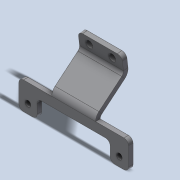
# Autodesk Inventor part: MuzzleHeadConnector2
Saved by Autodesk Inventor 2020 (Build 240168000, 168)
## iProperties
Created: 2021-07-22
Part Number: MuzzleHeadConnector2
Material: Generic
Document SubType Name: Sheet Metal
Designer: Val
Density: 1 g/cm^3
Sheet Metal Rule: Default
Appearance: Default
Flat Pattern Width: 5.75592 cm
Flat Pattern Length: 7.62 cm
Flat Pattern Area: 43.8601 cm^2
Sheet Metal Width: 2.266 in
Sheet Metal Length: 3.000 in
Sheet Metal Area: 6.798 in^2
Author: Val
Autodesk Inventor part; units mm, degrees
ref_plane "YZ Plane" through (0, 0, 0) normal (1, 0, 0) x (0, 1, 0)
ref_plane "XZ Plane" through (0, 0, 0) normal (0, 1, 0) x (-1, 0, 0)
ref_plane "XY Plane" through (0, 0, 0) normal (0, 0, 1) x (1, 0, 0)
sketch "Base" plane through (0, 0, 0) normal (0, 0, 1) x (1, 0, 0)
  line L0 (-38.1, 19.05) -> (38.1, 19.05)
  line L1 (38.1, 19.05) -> (38.1, 0)
  line L2 (38.1, 0) -> (-38.1, 0)
  line L3 (-38.1, 0) -> (-38.1, 19.05)
  line L4 (0, -3.81) -> (0, 22.86) construction
  line L5 (-25.4, 0) -> (-25.4, 12.7)
  line L6 (-25.4, 12.7) -> (25.4, 12.7)
  line L7 (25.4, 12.7) -> (25.4, 0)
  line L8 (-25.4, 12.7) -> (-38.1, 0) construction
  circle A0 centre (-31.75, 6.35) radius 2
  circle A1 centre (31.75, 6.35) radius 2
  point P0 (0, 0)
  point P1 (0, 19.05)
  dimension "d1" = 76.2
  dimension "d3" = 19.05
  dimension "d5" = 12.7
  dimension "d6" = 12.7
  dimension "d8" = 6.35
  dimension "d9" = 4
  measures "d1" distance of L0.start L0.end
  measures "d3" distance of L0.end L1.end
  measures "d5" distance between parallel lines of L3 L5
  measures "d6" distance between parallel lines of L1 L7
  measures "d8" distance between parallel lines of L0 L6
  measures "d9" diameter of A0
extrude "Plate1" add sketch "Base" along normal blind 3.175 contours L0 L1 L2 L7 L6 L5 L3
sketch "Sketch2" plane through (38.1, 21.4928, -1.1469) normal (0, 0.7693996, 0.6387678) x (-1, 0, 0)
  line L0 (76.2, 0) -> (0, 0)
  line L1 (0, 0) -> (0, -22.4187)
  line L2 (0, -22.4187) -> (76.2, -22.4187)
  line L3 (76.2, -22.4187) -> (76.2, 0)
  constraints: 6 end point, 1 horizontal, 1 perpendicular, 1 vertical
edge flange "MiddleFlangeFeature" height 25.4 angle 50.3 thickness 3.175 bend radius 3.175 thickness toward (0, 0.7693996, 0.6387678) relief straight relief width 3.175 relief depth 1.5875 edges at (0, 19.05, 0) wall of the first edge with corners at (-38.1, 21.4928, -1.1469) (38.1, 21.4928, -1.1469) (38.1, 35.8132, -18.3958) (-38.1, 35.8132, -18.3958)
bend "Bend1"
corner "Corner1"
sketch "Sketch3" plane through (38.1, 38.256, -16.3677) normal (0, 0.1166707, -0.9931706) x (-1, 0, 0)
  line L0 (76.2, 0) -> (0, 0)
  line L1 (0, 0) -> (0, -10.9761)
  line L2 (0, -10.9761) -> (76.2, -10.9761)
  line L3 (76.2, -10.9761) -> (76.2, 0)
  constraints: 6 end point, 1 horizontal, 1 perpendicular, 1 vertical
edge flange "MountFlangeFeature" height 12.7 angle -57 thickness 3.175 bend radius 3.175 thickness toward (0, 0.1166707, -0.9931706) relief straight relief width 3.175 relief depth 1.5875 edges at (0, 35.8132, -18.3958) wall of the first edge with corners at (-38.1, 38.256, -16.3677) (38.1, 38.256, -16.3677) (38.1, 49.1572, -15.0872) (-38.1, 49.1572, -15.0872)
bend "Bend2"
corner "Corner2"
sketch "TaperCut" plane through (0, 0, 3.175) normal (0, 0, 1) x (1, 0, 0)
  line L0 (-38.1, 19.05) -> (-38.1, 0) projected
  line L1 (-38.1, 19.05) -> (-15.24, 19.05)
  line L2 (-38.1, 19.05) -> (38.1, 19.05) projected
  line L3 (-15.24, 19.05) -> (-15.24, 49.1572)
  line L4 (-38.1, 39.9681) -> (-38.1, 49.1572) construction
  line L5 (-38.1, 49.1572) -> (38.1, 49.1572) projected
  line L6 (-38.1, 0) -> (-38.1, 19.05) projected
  line L7 (-38.1, 49.1572) -> (-38.1, 19.05)
  point P0 (0, 0)
  dimension "d35" = 22.86
  constraints: 6 end point, 2 point on line, 1 vertical
  measures "d35" distance between parallel lines of L4 L3
cut across bends "TaperCutFeature" sketch "TaperCut" k factor 0.44
mirror "TaperCutMirrorFeature" about plane through (0, 0, 0) normal (1, 0, 0) of "TaperCutFeature"
sketch "MountCut" plane through (-38.1, 49.1572, -15.0872) normal (0, -0.1166707, 0.9931706) x (1, 0, 0)
  line L0 (0, -8.402) -> (22.86, -8.402) projected
  line L1 (0, -8.402) -> (0, 0) projected
  line L2 (22.86, -8.402) -> (0, -8.402)
  line L3 (0, -8.402) -> (0, 0)
  line L4 (0, 0) -> (22.86, 0)
  line L5 (22.86, 0) -> (22.86, -8.402)
  line L6 (53.34, -8.402) -> (53.34, -9.2522) projected
  line L7 (53.34, -8.402) -> (76.2, -8.402)
  line L8 (76.2, -8.402) -> (76.2, 0)
  line L9 (76.2, 0) -> (53.34, 0)
  line L10 (53.34, 0) -> (53.34, -8.402)
  point P0 (38.1, -47.0612)
  constraints: 16 end point, 4 parallel, 2 horizontal, 2 perpendicular
extrude "MountCutFeature" cut sketch "MountCut" against normal blind 3.175
fillet "FilletsFeature" radius 3.175 10 edges at (-15.24, 49.3424, -16.6638) (15.24, 49.3424, -16.6638) (-38.1, 19.05, 1.5875) (-38.1, 0, 1.5875) (38.1, 19.05, 1.5875) (38.1, 0, 1.5875) (25.4, 0, 1.5875) (25.4, 12.7, 1.5875) (-25.4, 0, 1.5875) (-25.4, 12.7, 1.5875)
sketch "MountHoles" plane through (-38.1, 49.1572, -15.0872) normal (0, -0.1166707, 0.9931706) x (1, 0, 0)
  line L0 (0, 0) -> (76.2, 0) projected
  line L1 (38.1, 0) -> (38.1, -9.2522) construction
  line L2 (0, -9.2522) -> (76.2, -9.2522) projected
  circle A0 centre (30.1, -4.6261) radius 2.5
  line L3 (30.1, -4.6261) -> (38.1, -4.6261) construction
  circle A1 centre (46.1, -4.6261) radius 2.5
  point P0 (38.1, -47.0612)
  dimension "d31" = 5
  dimension "d32" = 8
  constraints: 4 end point, 3 midpoint, 2 centre point, 1 symmetric about line, 1 other
  measures "d31" diameter of A0
  measures "d32" distance from line of L1 L3.start
hole "MountHolesFeature" at (-8, 44.5627, -15.6269) at (8, 44.5627, -15.6269) direction (0, 0.1166707, -0.9931706) diameter 5 end through all
equation "\"d6\" = d5"
equation "\"d36\" = Thickness"
equation "\"d38\" = Thickness"
equation "\"d46\" = Thickness"
equation "\"d10\" = Thickness"
equation "\"d11\" = BendReliefWidth"
equation "\"d12\" = BendReliefDepth"
equation "\"d13\" = MinimumRemnant"
equation "\"d14\" = TransitionRadius"
equation "\"d17\" = BendRadius"
equation "\"d18\" = CornerReliefSize"
equation "\"d19\" = GapSize"
equation "\"d20\" = JacobiRadiusSize"
equation "\"d21\" = BendReliefWidth"
equation "\"d22\" = BendReliefDepth"
equation "\"d23\" = MinimumRemnant"
equation "\"d24\" = TransitionRadius"
equation "\"d27\" = BendRadius"
equation "\"d28\" = CornerReliefSize"
equation "\"d29\" = GapSize"
equation "\"d30\" = JacobiRadiusSize"
equation "\"BendRadius\" = Thickness"
equation "\"BendReliefWidth\" = Thickness"
equation "\"BendReliefDepth\" = 0.5 * Thickness"
equation "\"CornerReliefSize\" = 4 * Thickness"
equation "\"MinimumRemnant\" = 2 * Thickness"
equation "\"TransitionRadius\" = BendRadius"
equation "\"JacobiRadiusSize\" = BendRadius"
equation "\"GapSize\" = Thickness"
equation "\"Thickness\" = 3.175"
body "Solid1"
